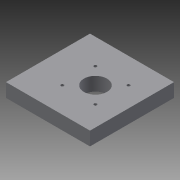
# Autodesk Inventor part: CNC-Z-axis- top plate
Saved by Autodesk Inventor 2015 (Build 190159000, 159)
## iProperties
Created: 2015-03-21
Part Number: CNC-Z-axis- top plate
Material: Generic
Document SubType Name: Modeling
Designer: Bangladesh
Density: 1 g/cm^3
Appearance: Default
Author: Bangladesh
Autodesk Inventor part; units mm, degrees
ref_plane "YZ Plane" through (0, 0, 0) normal (1, 0, 0) x (0, 1, 0)
ref_plane "XZ Plane" through (0, 0, 0) normal (0, 1, 0) x (-1, 0, 0)
ref_plane "XY Plane" through (0, 0, 0) normal (0, 0, 1) x (1, 0, 0)
sketch "Sketch1" plane through (0, 0, 0) normal (0, 1, 0) x (-1, 0, 0)
  line L0 (40, 40) -> (-40, 40)
  line L1 (-40, 40) -> (-40, -40)
  line L2 (-40, -40) -> (40, -40)
  line L3 (40, -40) -> (40, 40)
  line L4 (40, 40) -> (-40, -40) construction
  line L5 (-40, 40) -> (40, -40) construction
  point P0 (0, 0)
  dimension "d0" = 80
  dimension "d1" = 80
  constraints: 12 end point, 2 midpoint, 2 parallel, 1 horizontal, 1 perpendicular
  measures "d0" distance of L1.end L2.end
  measures "d1" distance of L0.end L1.end
extrude "Extrusion1" add sketch "Sketch1" along normal mid plane 13
sketch "Sketch2" plane through (0, 6.5, 0) normal (0, 1, 0) x (1, 0, 0)
  line L0 (-10.575, -15.76) -> (20.945, -15.76)
  line L1 (20.945, -15.76) -> (20.945, 15.76)
  line L2 (20.945, 15.76) -> (-10.575, 15.76)
  line L3 (-10.575, 15.76) -> (-10.575, -15.76)
  line L4 (-10.575, -15.76) -> (20.945, 15.76) construction
  line L5 (20.945, -15.76) -> (-10.575, 15.76) construction
  line L6 (-40, 40) -> (-40, -40) projected
  circle A0 centre (20.945, 15.76) radius 1.3891
  circle A1 centre (20.945, -15.76) radius 1.3891
  circle A2 centre (-10.575, 15.76) radius 1.3891
  circle A3 centre (-10.575, -15.76) radius 1.3891
  circle A4 centre (5.185, 0) radius 11
  point P0 (0, 0)
  dimension "d4" = 31.52
  dimension "d5" = 31.52
  dimension "d6" = 29.425
  dimension "d7" = 2.7781
  dimension "d8" = 2.7781
  dimension "d9" = 2.7781
  dimension "d10" = 2.7781
  dimension "d18" = 22
  constraints: 12 end point, 5 centre point, 3 coincident, 2 midpoint, 2 parallel, 1 horizontal, 1 perpendicular, 1 point on line
  measures "d4" distance of L1.end L2.end
  measures "d5" distance of L2.end L0.start
  measures "d6" distance between parallel lines of L6 L3
  measures "d7" diameter of A0
  measures "d8" diameter of A1
  measures "d9" diameter of A2
  measures "d10" diameter of A3
  measures "d18" diameter of A4
hole "Hole1" at (20.945, 6.5, -15.76) at (20.945, 6.5, 15.76) at (-10.575, 6.5, 15.76) at (-10.575, 6.5, -15.76) direction (0, -1, 0) diameter 2.7781 end through all
sketch "Sketch3" plane through (0, 6.5, 0) normal (0, 1, 0) x (1, 0, 0)
  line L0 (20.945, 15.76) -> (-10.575, 15.76)
  line L1 (-10.575, 15.76) -> (-10.575, -15.76)
  line L2 (-10.575, -15.76) -> (20.945, -15.76)
  line L3 (20.945, -15.76) -> (20.945, 15.76)
  line L4 (20.945, 15.76) -> (-10.575, -15.76) construction
  line L5 (-10.575, 15.76) -> (20.945, -15.76) construction
  line L6 (-40, 40) -> (-40, -40) projected
  circle A0 centre (5.185, 0) radius 11
  point P0 (0, 0)
  point P1 (5.185, 0)
  dimension "d19" = 31.52
  dimension "d20" = 31.52
  dimension "d21" = 29.425
  dimension "d22" = 22
  constraints: 12 end point, 4 midpoint, 2 parallel, 1 centre point, 1 horizontal, 1 perpendicular
  measures "d19" distance of L1.end L2.end
  measures "d20" distance of L0.end L1.end
  measures "d21" distance between parallel lines of L6 L1
  measures "d22" diameter of A0
hole "Hole2" at (5.185, 6.5, 0) direction (0, -1, 0) diameter 22 end through all
body "Solid1"
